Autodesk Fusion 360 part; units mm, degrees
(part 2 of 11)
  spline S13 degree 5 poles (-14.6436, -12.9958) (-14.6439, -12.9989) (-14.6444, -13.005) (-14.6453, -13.0142) (-14.6463, -13.0265) (-14.6476, -13.0418) (-14.6488, -13.0571) (-14.6499, -13.0724) (-14.6509, -13.0877) (-14.6519, -13.1029) (-14.6528, -13.1182) (-14.6536, -13.1334) (-14.6544, -13.1486) (-14.6551, -13.1638) (-14.6557, -13.1789) (-14.6562, -13.194) (-14.6567, -13.2091) (-14.6571, -13.2242) (-14.6574, -13.2393) (-14.6577, -13.2543) (-14.6579, -13.2693) (-14.658, -13.2843) (-14.658, -13.2993) (-14.658, -13.3142) (-14.6578, -13.3291) (-14.6577, -13.344) (-14.6574, -13.3589) (-14.657, -13.3737) (-14.6566, -13.3886) (-14.6561, -13.4033) (-14.6555, -13.4181) (-14.6549, -13.4328) (-14.6541, -13.4475) (-14.6533, -13.4622) (-14.6524, -13.4768) (-14.6514, -13.4915) (-14.6504, -13.506) (-14.6492, -13.5206) (-14.648, -13.5351) (-14.6467, -13.5496) (-14.6453, -13.564) (-14.6438, -13.5785) (-14.6422, -13.5928) (-14.6405, -13.6072) (-14.6388, -13.6215) (-14.637, -13.6358) (-14.635, -13.65) (-14.633, -13.6642) (-14.6309, -13.6784) (-14.6287, -13.6925) (-14.6264, -13.7066) (-14.624, -13.7206) (-14.6215, -13.7346) (-14.6188, -13.7486) (-14.6161, -13.7625) (-14.6133, -13.7763) (-14.6103, -13.7902) (-14.6073, -13.8039) (-14.6042, -13.8177) (-14.601, -13.8313) (-14.5976, -13.8449) (-14.5941, -13.8585) (-14.5903, -13.8719) (-14.5865, -13.8853) (-14.5825, -13.8986) (-14.5783, -13.9119) (-14.5741, -13.9251) (-14.5699, -13.9383) (-14.5654, -13.9514) (-14.5608, -13.9644) (-14.5558, -13.9772) (-14.5515, -13.9873) (-14.5479, -13.9947) (-14.5455, -13.9996) (-14.5442, -14.0021) knots -1 -1 -1 -1 -1 -1 -0.98571429 -0.97142857 -0.95714286 -0.94285714 -0.92857143 -0.91428571 -0.9 -0.88571429 -0.87142857 -0.85714286 -0.84285714 -0.82857143 -0.81428571 -0.8 -0.78571429 -0.77142857 -0.75714286 -0.74285714 -0.72857143 -0.71428571 -0.7 -0.68571429 -0.67142857 -0.65714286 -0.64285714 -0.62857143 -0.61428571 -0.6 -0.58571429 -0.57142857 -0.55714286 -0.54285714 -0.52857143 -0.51428571 -0.5 -0.48571429 -0.47142857 -0.45714286 -0.44285714 -0.42857143 -0.41428571 -0.4 -0.38571429 -0.37142857 -0.35714286 -0.34285714 -0.32857143 -0.31428571 -0.3 -0.28571429 -0.27142857 -0.25714286 -0.24285714 -0.22857143 -0.21428571 -0.2 -0.18571429 -0.17142857 -0.15714286 -0.14285714 -0.12857143 -0.11428571 -0.1 -0.08571429 -0.07142857 -0.05714286 -0.04285714 -0.02857143 -0.01428571 0 0 0 0 0 0
  line L13 (-14.5442, -14.0021) -> (-14.5127, -14.0629)
  arc A27 (-14.6099, -14.3947) -> (-14.5127, -14.0629) centre (-14.7346, -14.178) ccw
  arc A28 (-14.6099, -14.3947) -> (-14.7093, -14.4532) centre (-11.6741, -19.5) ccw
  arc A29 (-15.0466, -14.3769) -> (-14.7093, -14.4532) centre (-14.8381, -14.2389) ccw
  line L14 (-15.0466, -14.3769) -> (-15.0844, -14.3198)
  spline S14 degree 5 poles (-15.0844, -14.3198) (-15.0859, -14.3175) (-15.089, -14.313) (-15.0938, -14.3062) (-15.1005, -14.2975) (-15.1093, -14.287) (-15.1184, -14.2766) (-15.1277, -14.2664) (-15.1371, -14.2562) (-15.1466, -14.2461) (-15.1562, -14.2361) (-15.1659, -14.2261) (-15.1757, -14.2162) (-15.1857, -14.2064) (-15.1958, -14.1968) (-15.206, -14.1872) (-15.2164, -14.1777) (-15.2269, -14.1683) (-15.2375, -14.159) (-15.2481, -14.1497) (-15.2589, -14.1405) (-15.2697, -14.1314) (-15.2806, -14.1223) (-15.2916, -14.1133) (-15.3027, -14.1044) (-15.3139, -14.0955) (-15.3252, -14.0867) (-15.3365, -14.078) (-15.3479, -14.0693) (-15.3594, -14.0607) (-15.371, -14.0522) (-15.3827, -14.0437) (-15.3944, -14.0353) (-15.4062, -14.0269) (-15.4181, -14.0186) (-15.4301, -14.0103) (-15.4421, -14.0022) (-15.4542, -13.994) (-15.4663, -13.9859) (-15.4786, -13.9779) (-15.4909, -13.97) (-15.5032, -13.9621) (-15.5156, -13.9542) (-15.5281, -13.9464) (-15.5407, -13.9387) (-15.5533, -13.931) (-15.566, -13.9234) (-15.5787, -13.9158) (-15.5915, -13.9083) (-15.6044, -13.9008) (-15.6173, -13.8934) (-15.6303, -13.8861) (-15.6433, -13.8788) (-15.6564, -13.8715) (-15.6696, -13.8643) (-15.6828, -13.8572) (-15.696, -13.8501) (-15.7093, -13.8431) (-15.7227, -13.8361) (-15.7362, -13.8292) (-15.7496, -13.8223) (-15.7632, -13.8155) (-15.7768, -13.8087) (-15.7904, -13.802) (-15.8041, -13.7953) (-15.8179, -13.7887) (-15.8317, -13.7822) (-15.8455, -13.7757) (-15.8594, -13.7692) (-15.8734, -13.7628) (-15.8874, -13.7564) (-15.8986, -13.7514) (-15.9071, -13.7476) (-15.9127, -13.7451) (-15.9156, -13.7439) knots 0 0 0 0 0 0 0.01428571 0.02857143 0.04285714 0.05714286 0.07142857 0.08571429 0.1 0.11428571 0.12857143 0.14285714 0.15714286 0.17142857 0.18571429 0.2 0.21428571 0.22857143 0.24285714 0.25714286 0.27142857 0.28571429 0.3 0.31428571 0.32857143 0.34285714 0.35714286 0.37142857 0.38571429 0.4 0.41428571 0.42857143 0.44285714 0.45714286 0.47142857 0.48571429 0.5 0.51428571 0.52857143 0.54285714 0.55714286 0.57142857 0.58571429 0.6 0.61428571 0.62857143 0.64285714 0.65714286 0.67142857 0.68571429 0.7 0.71428571 0.72857143 0.74285714 0.75714286 0.77142857 0.78571429 0.8 0.81428571 0.82857143 0.84285714 0.85714286 0.87142857 0.88571429 0.9 0.91428571 0.92857143 0.94285714 0.95714286 0.97142857 0.98571429 1 1 1 1 1 1
  arc A30 (-15.9156, -13.7439) -> (-16.2258, -13.986) centre (-11.6741, -19.5) ccw
  spline S15 degree 5 poles (-16.2258, -13.986) (-16.2253, -13.989) (-16.2243, -13.9951) (-16.2227, -14.0042) (-16.2205, -14.0163) (-16.2178, -14.0315) (-16.2149, -14.0466) (-16.2121, -14.0616) (-16.2091, -14.0766) (-16.2061, -14.0916) (-16.203, -14.1066) (-16.1999, -14.1215) (-16.1967, -14.1363) (-16.1934, -14.1512) (-16.1901, -14.166) (-16.1867, -14.1807) (-16.1833, -14.1954) (-16.1798, -14.2101) (-16.1762, -14.2247) (-16.1725, -14.2393) (-16.1688, -14.2539) (-16.165, -14.2684) (-16.1612, -14.2829) (-16.1573, -14.2973) (-16.1533, -14.3117) (-16.1493, -14.326) (-16.1452, -14.3403) (-16.141, -14.3545) (-16.1367, -14.3687) (-16.1324, -14.3829) (-16.128, -14.397) (-16.1236, -14.411) (-16.1191, -14.425) (-16.1145, -14.439) (-16.1098, -14.4529) (-16.1051, -14.4668) (-16.1003, -14.4806) (-16.0954, -14.4943) (-16.0905, -14.508) (-16.0855, -14.5217) (-16.0804, -14.5353) (-16.0752, -14.5488) (-16.07, -14.5623) (-16.0646, -14.5757) (-16.0592, -14.5891) (-16.0538, -14.6024) (-16.0482, -14.6157) (-16.0426, -14.6289) (-16.0369, -14.642) (-16.0311, -14.6551) (-16.0252, -14.6681) (-16.0193, -14.681) (-16.0132, -14.6939) (-16.0071, -14.7067) (-16.0008, -14.7194) (-15.9945, -14.7321) (-15.9881, -14.7447) (-15.9816, -14.7572) (-15.9751, -14.7696) (-15.9684, -14.782) (-15.9616, -14.7943) (-15.9547, -14.8064) (-15.9476, -14.8185) (-15.9404, -14.8304) (-15.9331, -14.8422) (-15.9257, -14.854) (-15.9182, -14.8656) (-15.9107, -14.8772) (-15.903, -14.8888) (-15.8952, -14.9001) (-15.887, -14.9112) (-15.8802, -14.9198) (-15.8749, -14.9261) (-15.8712, -14.9302) (-15.8694, -14.9322) knots -1 -1 -1 -1 -1 -1 -0.98571429 -0.97142857 -0.95714286 -0.94285714 -0.92857143 -0.91428571 -0.9 -0.88571429 -0.87142857 -0.85714286 -0.84285714 -0.82857143 -0.81428571 -0.8 -0.78571429 -0.77142857 -0.75714286 -0.74285714 -0.72857143 -0.71428571 -0.7 -0.68571429 -0.67142857 -0.65714286 -0.64285714 -0.62857143 -0.61428571 -0.6 -0.58571429 -0.57142857 -0.55714286 -0.54285714 -0.52857143 -0.51428571 -0.5 -0.48571429 -0.47142857 -0.45714286 -0.44285714 -0.42857143 -0.41428571 -0.4 -0.38571429 -0.37142857 -0.35714286 -0.34285714 -0.32857143 -0.31428571 -0.3 -0.28571429 -0.27142857 -0.25714286 -0.24285714 -0.22857143 -0.21428571 -0.2 -0.18571429 -0.17142857 -0.15714286 -0.14285714 -0.12857143 -0.11428571 -0.1 -0.08571429 -0.07142857 -0.05714286 -0.04285714 -0.02857143 -0.01428571 0 0 0 0 0 0
  line L15 (-15.8694, -14.9322) -> (-15.8232, -14.9828)
  arc A31 (-15.8312, -15.3285) -> (-15.8232, -14.9828) centre (-16.0077, -15.1515) ccw
  arc A32 (-15.8312, -15.3285) -> (-15.9121, -15.4107) centre (-11.6741, -19.5) ccw
  arc A33 (-16.2576, -15.4243) -> (-15.9121, -15.4107) centre (-16.092, -15.2371) ccw
  line L16 (-16.2576, -15.4243) -> (-16.3089, -15.3789)
  spline S16 degree 5 poles (-16.3089, -15.3789) (-16.311, -15.3771) (-16.3151, -15.3735) (-16.3215, -15.3683) (-16.3302, -15.3616) (-16.3415, -15.3537) (-16.3529, -15.346) (-16.3646, -15.3385) (-16.3763, -15.3312) (-16.3881, -15.3239) (-16.4, -15.3167) (-16.4119, -15.3095) (-16.424, -15.3025) (-16.4361, -15.2957) (-16.4484, -15.2889) (-16.4608, -15.2823) (-16.4732, -15.2759) (-16.4858, -15.2695) (-16.4984, -15.2632) (-16.5111, -15.257) (-16.5238, -15.2509) (-16.5367, -15.2449) (-16.5496, -15.239) (-16.5625, -15.2331) (-16.5755, -15.2274) (-16.5886, -15.2217) (-16.6018, -15.2161) (-16.615, -15.2106) (-16.6283, -15.2052) (-16.6417, -15.1999) (-16.6551, -15.1946) (-16.6685, -15.1894) (-16.682, -15.1843) (-16.6956, -15.1793) (-16.7092, -15.1744) (-16.7229, -15.1695) (-16.7366, -15.1647) (-16.7504, -15.16) (-16.7643, -15.1553) (-16.7781, -15.1508) (-16.7921, -15.1462) (-16.8061, -15.1418) (-16.8201, -15.1374) (-16.8342, -15.1332) (-16.8483, -15.1289) (-16.8625, -15.1248) (-16.8767, -15.1207) (-16.891, -15.1167) (-16.9053, -15.1127) (-16.9196, -15.1089) (-16.934, -15.105) (-16.9485, -15.1013) (-16.9629, -15.0976) (-16.9775, -15.094) (-16.992, -15.0905) (-17.0066, -15.087) (-17.0213, -15.0836) (-17.036, -15.0802) (-17.0507, -15.077) (-17.0655, -15.0737) (-17.0803, -15.0706) (-17.0951, -15.0675) (-17.11, -15.0645) (-17.1249, -15.0615) (-17.1399, -15.0586) (-17.1549, -15.0558) (-17.1699, -15.053) (-17.185, -15.0503) (-17.2001, -15.0477) (-17.2152, -15.0451) (-17.2304, -15.0426) (-17.2425, -15.0407) (-17.2517, -15.0392) (-17.2578, -15.0383) (-17.2608, -15.0378) knots 0 0 0 0 0 0 0.01428571 0.02857143 0.04285714 0.05714286 0.07142857 0.08571429 0.1 0.11428571 0.12857143 0.14285714 0.15714286 0.17142857 0.18571429 0.2 0.21428571 0.22857143 0.24285714 0.25714286 0.27142857 0.28571429 0.3 0.31428571 0.32857143 0.34285714 0.35714286 0.37142857 0.38571429 0.4 0.41428571 0.42857143 0.44285714 0.45714286 0.47142857 0.48571429 0.5 0.51428571 0.52857143 0.54285714 0.55714286 0.57142857 0.58571429 0.6 0.61428571 0.62857143 0.64285714 0.65714286 0.67142857 0.68571429 0.7 0.71428571 0.72857143 0.74285714 0.75714286 0.77142857 0.78571429 0.8 0.81428571 0.82857143 0.84285714 0.85714286 0.87142857 0.88571429 0.9 0.91428571 0.92857143 0.94285714 0.95714286 0.97142857 0.98571429 1 1 1 1 1 1
  arc A34 (-17.2608, -15.0378) -> (-17.4979, -15.3519) centre (-11.6741, -19.5) ccw
  spline S17 degree 5 poles (-17.4979, -15.3519) (-17.4966, -15.3547) (-17.494, -15.3603) (-17.4901, -15.3687) (-17.4849, -15.3799) (-17.4783, -15.3938) (-17.4717, -15.4076) (-17.465, -15.4214) (-17.4583, -15.4352) (-17.4515, -15.4489) (-17.4446, -15.4625) (-17.4378, -15.4761) (-17.4308, -15.4896) (-17.4238, -15.5031) (-17.4168, -15.5165) (-17.4097, -15.5299) (-17.4026, -15.5432) (-17.3954, -15.5565) (-17.3881, -15.5697) (-17.3808, -15.5829) (-17.3735, -15.5959) (-17.3661, -15.609) (-17.3586, -15.622) (-17.3511, -15.6349) (-17.3435, -15.6477) (-17.3359, -15.6605) (-17.3283, -15.6733) (-17.3205, -15.6859) (-17.3128, -15.6986) (-17.3049, -15.7111) (-17.297, -15.7236) (-17.2891, -15.736) (-17.2811, -15.7484) (-17.2731, -15.7607) (-17.265, -15.7729) (-17.2568, -15.7851) (-17.2486, -15.7972) (-17.2403, -15.8092) (-17.232, -15.8212) (-17.2236, -15.8331) (-17.2152, -15.8449) (-17.2067, -15.8566) (-17.1981, -15.8683) (-17.1895, -15.8799) (-17.1809, -15.8914) (-17.1721, -15.9028) (-17.1633, -15.9142) (-17.1545, -15.9255) (-17.1456, -15.9367) (-17.1366, -15.9478) (-17.1276, -15.9589) (-17.1184, -15.9698) (-17.1093, -15.9807) (-17.1, -15.9915) (-17.0907, -16.0021) (-17.0813, -16.0127) (-17.0719, -16.0232) (-17.0624, -16.0336) (-17.0528, -16.044) (-17.0432, -16.0542) (-17.0335, -16.0643) (-17.0236, -16.0742) (-17.0137, -16.084) (-17.0036, -16.0937) (-16.9935, -16.1032) (-16.9833, -16.1126) (-16.9731, -16.122) (-16.9628, -16.1313) (-16.9524, -16.1404) (-16.9419, -16.1493) (-16.9312, -16.158) (-16.9223, -16.1645) (-16.9156, -16.1692) (-16.911, -16.1722) (-16.9087, -16.1737) knots -1 -1 -1 -1 -1 -1 -0.98571429 -0.97142857 -0.95714286 -0.94285714 -0.92857143 -0.91428571 -0.9 -0.88571429 -0.87142857 -0.85714286 -0.84285714 -0.82857143 -0.81428571 -0.8 -0.78571429 -0.77142857 -0.75714286 -0.74285714 -0.72857143 -0.71428571 -0.7 -0.68571429 -0.67142857 -0.65714286 -0.64285714 -0.62857143 -0.61428571 -0.6 -0.58571429 -0.57142857 -0.55714286 -0.54285714 -0.52857143 -0.51428571 -0.5 -0.48571429 -0.47142857 -0.45714286 -0.44285714 -0.42857143 -0.41428571 -0.4 -0.38571429 -0.37142857 -0.35714286 -0.34285714 -0.32857143 -0.31428571 -0.3 -0.28571429 -0.27142857 -0.25714286 -0.24285714 -0.22857143 -0.21428571 -0.2 -0.18571429 -0.17142857 -0.15714286 -0.14285714 -0.12857143 -0.11428571 -0.1 -0.08571429 -0.07142857 -0.05714286 -0.04285714 -0.02857143 -0.01428571 0 0 0 0 0 0
  line L17 (-16.9087, -16.1737) -> (-16.8509, -16.2106)
  arc A35 (-16.7692, -16.5466) -> (-16.8509, -16.2106) centre (-16.9855, -16.4212) ccw
  arc A36 (-16.7692, -16.5466) -> (-16.8261, -16.6469) centre (-11.6741, -19.5) ccw
  arc A37 (-17.1563, -16.7495) -> (-16.8261, -16.6469) centre (-17.0448, -16.5258) ccw
  line L18 (-17.1563, -16.7495) -> (-17.2176, -16.7189)
  spline S18 degree 5 poles (-17.2176, -16.7189) (-17.2201, -16.7177) (-17.225, -16.7153) (-17.2325, -16.7119) (-17.2427, -16.7077) (-17.2556, -16.7029) (-17.2687, -16.6985) (-17.2818, -16.6943) (-17.2951, -16.6902) (-17.3083, -16.6863) (-17.3217, -16.6823) (-17.3351, -16.6785) (-17.3485, -16.6749) (-17.362, -16.6714) (-17.3756, -16.6681) (-17.3893, -16.6649) (-17.403, -16.6619) (-17.4168, -16.659) (-17.4306, -16.6562) (-17.4444, -16.6535) (-17.4583, -16.6509) (-17.4723, -16.6484) (-17.4863, -16.646) (-17.5003, -16.6437) (-17.5144, -16.6415) (-17.5285, -16.6395) (-17.5426, -16.6375) (-17.5568, -16.6356) (-17.5711, -16.6338) (-17.5854, -16.6321) (-17.5997, -16.6305) (-17.614, -16.629) (-17.6284, -16.6275) (-17.6428, -16.6262) (-17.6572, -16.6249) (-17.6717, -16.6238) (-17.6862, -16.6227) (-17.7007, -16.6217) (-17.7153, -16.6208) (-17.7299, -16.62) (-17.7445, -16.6192) (-17.7592, -16.6186) (-17.7739, -16.618) (-17.7886, -16.6175) (-17.8033, -16.617) (-17.8181, -16.6167) (-17.8329, -16.6164) (-17.8477, -16.6162) (-17.8625, -16.6161) (-17.8774, -16.6161) (-17.8923, -16.6162) (-17.9072, -16.6163) (-17.9221, -16.6165) (-17.9371, -16.6167) (-17.9521, -16.6171) (-17.9671, -16.6175) (-17.9821, -16.618) (-17.9972, -16.6186) (-18.0123, -16.6192) (-18.0274, -16.6199) (-18.0425, -16.6207) (-18.0576, -16.6216) (-18.0728, -16.6225) (-18.0879, -16.6235) (-18.1031, -16.6246) (-18.1184, -16.6258) (-18.1336, -16.627) (-18.1488, -16.6283) (-18.1641, -16.6296) (-18.1794, -16.6311) (-18.1947, -16.6326) (-18.207, -16.6338) (-18.2162, -16.6348) (-18.2223, -16.6355) (-18.2254, -16.6358) knots 0 0 0 0 0 0 0.01428571 0.02857143 0.04285714 0.05714286 0.07142857 0.08571429 0.1 0.11428571 0.12857143 0.14285714 0.15714286 0.17142857 0.18571429 0.2 0.21428571 0.22857143 0.24285714 0.25714286 0.27142857 0.28571429 0.3 0.31428571 0.32857143 0.34285714 0.35714286 0.37142857 0.38571429 0.4 0.41428571 0.42857143 0.44285714 0.45714286 0.47142857 0.48571429 0.5 0.51428571 0.52857143 0.54285714 0.55714286 0.57142857 0.58571429 0.6 0.61428571 0.62857143 0.64285714 0.65714286 0.67142857 0.68571429 0.7 0.71428571 0.72857143 0.74285714 0.75714286 0.77142857 0.78571429 0.8 0.81428571 0.82857143 0.84285714 0.85714286 0.87142857 0.88571429 0.9 0.91428571 0.92857143 0.94285714 0.95714286 0.97142857 0.98571429 1 1 1 1 1 1
  arc A38 (-18.2254, -16.6358) -> (-18.373, -17.0005) centre (-11.6741, -19.5) ccw
  spline S19 degree 5 poles (-18.373, -17.0005) (-18.3711, -17.0029) (-18.3671, -17.0077) (-18.3612, -17.0148) (-18.3532, -17.0242) (-18.3433, -17.0359) (-18.3333, -17.0476) (-18.3233, -17.0592) (-18.3132, -17.0707) (-18.3031, -17.0822) (-18.293, -17.0936) (-18.2828, -17.1049) (-18.2726, -17.1162) (-18.2624, -17.1274) (-18.2521, -17.1386) (-18.2418, -17.1497) (-18.2314, -17.1607) (-18.2211, -17.1716) (-18.2106, -17.1825) (-18.2002, -17.1933) (-18.1897, -17.2041) (-18.1792, -17.2147) (-18.1686, -17.2253) (-18.158, -17.2359) (-18.1474, -17.2463) (-18.1367, -17.2567) (-18.126, -17.2671) (-18.1153, -17.2773) (-18.1045, -17.2875) (-18.0937, -17.2976) (-18.0829, -17.3076) (-18.072, -17.3175) (-18.0611, -17.3274) (-18.0501, -17.3372) (-18.0391, -17.3469) (-18.0281, -17.3566) (-18.017, -17.3661) (-18.0059, -17.3756) (-17.9948, -17.385) (-17.9836, -17.3943) (-17.9724, -17.4036) (-17.9612, -17.4127) (-17.9499, -17.4218) (-17.9385, -17.4307) (-17.9272, -17.4396) (-17.9158, -17.4484) (-17.9044, -17.4571) (-17.8929, -17.4657) (-17.8814, -17.4742) (-17.8698, -17.4827) (-17.8582, -17.491) (-17.8466, -17.4992) (-17.8349, -17.5073) (-17.8232, -17.5153) (-17.8115, -17.5232) (-17.7997, -17.531) (-17.7878, -17.5387) (-17.7759, -17.5463) (-17.764, -17.5538) (-17.7521, -17.5612) (-17.7401, -17.5685) (-17.728, -17.5755) (-17.7159, -17.5824) (-17.7037, -17.5891) (-17.6914, -17.5957) (-17.6791, -17.6022) (-17.6668, -17.6086) (-17.6545, -17.6148) (-17.6421, -17.621) (-17.6296, -17.6269) (-17.617, -17.6325) (-17.6068, -17.6365) (-17.599, -17.6393) (-17.5938, -17.641) (-17.5912, -17.6418) knots -1 -1 -1 -1 -1 -1 -0.98571429 -0.97142857 -0.95714286 -0.94285714 -0.92857143 -0.91428571 -0.9 -0.88571429 -0.87142857 -0.85714286 -0.84285714 -0.82857143 -0.81428571 -0.8 -0.78571429 -0.77142857 -0.75714286 -0.74285714 -0.72857143 -0.71428571 -0.7 -0.68571429 -0.67142857 -0.65714286 -0.64285714 -0.62857143 -0.61428571 -0.6 -0.58571429 -0.57142857 -0.55714286 -0.54285714 -0.52857143 -0.51428571 -0.5 -0.48571429 -0.47142857 -0.45714286 -0.44285714 -0.42857143 -0.41428571 -0.4 -0.38571429 -0.37142857 -0.35714286 -0.34285714 -0.32857143 -0.31428571 -0.3 -0.28571429 -0.27142857 -0.25714286 -0.24285714 -0.22857143 -0.21428571 -0.2 -0.18571429 -0.17142857 -0.15714286 -0.14285714 -0.12857143 -0.11428571 -0.1 -0.08571429 -0.07142857 -0.05714286 -0.04285714 -0.02857143 -0.01428571 0 0 0 0 0 0
  line L19 (-17.5912, -17.6418) -> (-17.5259, -17.6625)
  arc A39 (-17.36, -17.966) -> (-17.5259, -17.6625) centre (-17.6014, -17.9008) ccw
  arc A40 (-17.36, -17.966) -> (-17.389, -18.0775) centre (-11.6741, -19.5) ccw
  arc A41 (-17.6814, -18.2621) -> (-17.389, -18.0775) centre (-17.6316, -18.0171) ccw
  line L20 (-17.6814, -18.2621) -> (-17.7485, -18.2485)
  spline S20 degree 5 poles (-17.7485, -18.2485) (-17.7512, -18.2479) (-17.7566, -18.2469) (-17.7647, -18.2455) (-17.7756, -18.2441) (-17.7893, -18.2428) (-17.8031, -18.2419) (-17.8169, -18.2413) (-17.8308, -18.2408) (-17.8446, -18.2404) (-17.8585, -18.24) (-17.8724, -18.2398) (-17.8863, -18.2398) (-17.9003, -18.2399) (-17.9143, -18.2402) (-17.9283, -18.2407) (-17.9423, -18.2414) (-17.9564, -18.2421) (-17.9705, -18.243) (-17.9845, -18.244) (-17.9986, -18.245) (-18.0128, -18.2462) (-18.0269, -18.2475) (-18.041, -18.249) (-18.0552, -18.2505) (-18.0694, -18.2521) (-18.0836, -18.2539) (-18.0978, -18.2558) (-18.112, -18.2577) (-18.1262, -18.2598) (-18.1404, -18.2619) (-18.1547, -18.2641) (-18.1689, -18.2665) (-18.1832, -18.2689) (-18.1975, -18.2714) (-18.2118, -18.2741) (-18.226, -18.2768) (-18.2403, -18.2796) (-18.2547, -18.2825) (-18.269, -18.2854) (-18.2833, -18.2885) (-18.2976, -18.2917) (-18.3119, -18.2949) (-18.3263, -18.2982) (-18.3406, -18.3016) (-18.355, -18.3051) (-18.3693, -18.3087) (-18.3837, -18.3123) (-18.3981, -18.3161) (-18.4124, -18.3199) (-18.4268, -18.3238) (-18.4412, -18.3278) (-18.4556, -18.3318) (-18.4699, -18.336) (-18.4843, -18.3402) (-18.4987, -18.3445) (-18.5131, -18.3488) (-18.5275, -18.3533) (-18.5419, -18.3578) (-18.5563, -18.3624) (-18.5707, -18.3671) (-18.5851, -18.3718) (-18.5995, -18.3767) (-18.6139, -18.3816) (-18.6283, -18.3865) (-18.6427, -18.3916) (-18.6571, -18.3967) (-18.6715, -18.4019) (-18.6859, -18.4072) (-18.7003, -18.4125) (-18.7147, -18.4179) (-18.7262, -18.4223) (-18.7348, -18.4256) (-18.7406, -18.4278) (-18.7435, -18.429) knots 0 0 0 0 0 0 0.01428571 0.02857143 0.04285714 0.05714286 0.07142857 0.08571429 0.1 0.11428571 0.12857143 0.14285714 0.15714286 0.17142857 0.18571429 0.2 0.21428571 0.22857143 0.24285714 0.25714286 0.27142857 0.28571429 0.3 0.31428571 0.32857143 0.34285714 0.35714286 0.37142857 0.38571429 0.4 0.41428571 0.42857143 0.44285714 0.45714286 0.47142857 0.48571429 0.5 0.51428571 0.52857143 0.54285714 0.55714286 0.57142857 0.58571429 0.6 0.61428571 0.62857143 0.64285714 0.65714286 0.67142857 0.68571429 0.7 0.71428571 0.72857143 0.74285714 0.75714286 0.77142857 0.78571429 0.8 0.81428571 0.82857143 0.84285714 0.85714286 0.87142857 0.88571429 0.9 0.91428571 0.92857143 0.94285714 0.95714286 0.97142857 0.98571429 1 1 1 1 1 1
  arc A42 (-18.7435, -18.429) -> (-18.7917, -18.8195) centre (-11.6741, -19.5) ccw
  spline S21 degree 5 poles (-18.7917, -18.8195) (-18.7892, -18.8213) (-18.7841, -18.8249) (-18.7766, -18.8302) (-18.7664, -18.8372) (-18.7538, -18.846) (-18.7411, -18.8547) (-18.7284, -18.8633) (-18.7157, -18.8718) (-18.703, -18.8803) (-18.6903, -18.8887) (-18.6775, -18.897) (-18.6647, -18.9053) (-18.652, -18.9134) (-18.6391, -18.9216) (-18.6263, -18.9296) (-18.6135, -18.9376) (-18.6006, -18.9454) (-18.5877, -18.9533) (-18.5748, -18.961) (-18.5619, -18.9687) (-18.549, -18.9762) (-18.536, -18.9838) (-18.5231, -18.9912) (-18.5101, -18.9985) (-18.4971, -19.0058) (-18.4841, -19.013) (-18.4711, -19.0201) (-18.458, -19.0272) (-18.445, -19.0341) (-18.4319, -19.041) (-18.4188, -19.0478) (-18.4057, -19.0545) (-18.3926, -19.0611) (-18.3795, -19.0677) (-18.3663, -19.0741) (-18.3532, -19.0805) (-18.34, -19.0868) (-18.3268, -19.093) (-18.3136, -19.0991) (-18.3004, -19.1051) (-18.2872, -19.111) (-18.2739, -19.1168) (-18.2607, -19.1226) (-18.2474, -19.1282) (-18.2341, -19.1338) (-18.2208, -19.1392) (-18.2075, -19.1446) (-18.1942, -19.1498) (-18.1808, -19.155) (-18.1675, -19.16) (-18.1541, -19.165) (-18.1407, -19.1698) (-18.1274, -19.1745) (-18.114, -19.1791) (-18.1005, -19.1835) (-18.0871, -19.1879) (-18.0737, -19.1922) (-18.0602, -19.1963) (-18.0468, -19.2004) (-18.0333, -19.2042) (-18.0198, -19.208) (-18.0063, -19.2115) (-17.9928, -19.2148) (-17.9792, -19.218) (-17.9657, -19.2211) (-17.9521, -19.224) (-17.9386, -19.2269) (-17.925, -19.2296) (-17.9115, -19.2321) (-17.8979, -19.2342) (-17.887, -19.2355) (-17.8787, -19.2362) (-17.8733, -19.2365) (-17.8705, -19.2366) knots -1 -1 -1 -1 -1 -1 -0.98571429 -0.97142857 -0.95714286 -0.94285714 -0.92857143 -0.91428571 -0.9 -0.88571429 -0.87142857 -0.85714286 -0.84285714 -0.82857143 -0.81428571 -0.8 -0.78571429 -0.77142857 -0.75714286 -0.74285714 -0.72857143 -0.71428571 -0.7 -0.68571429 -0.67142857 -0.65714286 -0.64285714 -0.62857143 -0.61428571 -0.6 -0.58571429 -0.57142857 -0.55714286 -0.54285714 -0.52857143 -0.51428571 -0.5 -0.48571429 -0.47142857 -0.45714286 -0.44285714 -0.42857143 -0.41428571 -0.4 -0.38571429 -0.37142857 -0.35714286 -0.34285714 -0.32857143 -0.31428571 -0.3 -0.28571429 -0.27142857 -0.25714286 -0.24285714 -0.22857143 -0.21428571 -0.2 -0.18571429 -0.17142857 -0.15714286 -0.14285714 -0.12857143 -0.11428571 -0.1 -0.08571429 -0.07142857 -0.05714286 -0.04285714 -0.02857143 -0.01428571 0 0 0 0 0 0
  line L21 (-17.8705, -19.2366) -> (-17.8021, -19.2397)
  arc A43 (-17.5633, -19.4898) -> (-17.8021, -19.2397) centre (-17.8133, -19.4894) ccw
  arc A44 (-17.5633, -19.4898) -> (-17.5624, -19.6051) centre (-11.6741, -19.5) ccw
  arc A45 (-17.7971, -19.8591) -> (-17.5624, -19.6051) centre (-17.8124, -19.6095) ccw
  line L22 (-17.7971, -19.8591) -> (-17.8655, -19.8633)
  spline S22 degree 5 poles (-17.8655, -19.8633) (-17.8682, -19.8634) (-17.8737, -19.8638) (-17.8819, -19.8646) (-17.8928, -19.8661) (-17.9063, -19.8684) (-17.9199, -19.8711) (-17.9334, -19.8741) (-17.9469, -19.8771) (-17.9604, -19.8803) (-17.9739, -19.8836) (-17.9874, -19.887) (-18.0008, -19.8906) (-18.0143, -19.8943) (-18.0277, -19.8982) (-18.0411, -19.9023) (-18.0545, -19.9066) (-18.0679, -19.9109) (-18.0813, -19.9154) (-18.0946, -19.92) (-18.1079, -19.9247) (-18.1213, -19.9295) (-18.1346, -19.9344) (-18.1479, -19.9395) (-18.1612, -19.9446) (-18.1744, -19.9499) (-18.1877, -19.9552) (-18.2009, -19.9607) (-18.2141, -19.9663) (-18.2273, -19.9719) (-18.2405, -19.9777) (-18.2537, -19.9835) (-18.2669, -19.9895) (-18.28, -19.9955) (-18.2932, -20.0017) (-18.3063, -20.0079) (-18.3194, -20.0142) (-18.3325, -20.0206) (-18.3455, -20.0271) (-18.3586, -20.0337) (-18.3716, -20.0404) (-18.3847, -20.0471) (-18.3977, -20.0539) (-18.4107, -20.0609) (-18.4236, -20.0679) (-18.4366, -20.075) (-18.4495, -20.0821) (-18.4625, -20.0894) (-18.4754, -20.0967) (-18.4883, -20.1041) (-18.5011, -20.1116) (-18.514, -20.1192) (-18.5268, -20.1268) (-18.5397, -20.1345) (-18.5525, -20.1423) (-18.5653, -20.1502) (-18.578, -20.1581) (-18.5908, -20.1661) (-18.6035, -20.1742) (-18.6162, -20.1824) (-18.6289, -20.1906) (-18.6416, -20.199) (-18.6543, -20.2073) (-18.6669, -20.2158) (-18.6795, -20.2243) (-18.6921, -20.2329) (-18.7047, -20.2416) (-18.7173, -20.2504) (-18.7298, -20.2592) (-18.7423, -20.2681) (-18.7548, -20.277) (-18.7648, -20.2842) (-18.7723, -20.2897) (-18.7773, -20.2933) (-18.7798, -20.2951) knots 0 0 0 0 0 0 0.01428571 0.02857143 0.04285714 0.05714286 0.07142857 0.08571429 0.1 0.11428571 0.12857143 0.14285714 0.15714286 0.17142857 0.18571429 0.2 0.21428571 0.22857143 0.24285714 0.25714286 0.27142857 0.28571429 0.3 0.31428571 0.32857143 0.34285714 0.35714286 0.37142857 0.38571429 0.4 0.41428571 0.42857143 0.44285714 0.45714286 0.47142857 0.48571429 0.5 0.51428571 0.52857143 0.54285714 0.55714286 0.57142857 0.58571429 0.6 0.61428571 0.62857143 0.64285714 0.65714286 0.67142857 0.68571429 0.7 0.71428571 0.72857143 0.74285714 0.75714286 0.77142857 0.78571429 0.8 0.81428571 0.82857143 0.84285714 0.85714286 0.87142857 0.88571429 0.9 0.91428571 0.92857143 0.94285714 0.95714286 0.97142857 0.98571429 1 1 1 1 1 1
  arc A46 (-18.7798, -20.2951) -> (-18.7253, -20.6848) centre (-11.6741, -19.5) ccw
  spline S23 degree 5 poles (-18.7253, -20.6848) (-18.7224, -20.6859) (-18.7166, -20.6881) (-18.7079, -20.6912) (-18.6963, -20.6954) (-18.6818, -20.7006) (-18.6674, -20.7057) (-18.6529, -20.7108) (-18.6384, -20.7157) (-18.6239, -20.7206) (-18.6094, -20.7254) (-18.595, -20.7302) (-18.5805, -20.7348) (-18.566, -20.7394) (-18.5515, -20.7439) (-18.5371, -20.7484) (-18.5226, -20.7527) (-18.5081, -20.757) (-18.4937, -20.7613) (-18.4792, -20.7654) (-18.4648, -20.7694) (-18.4503, -20.7734) (-18.4359, -20.7773) (-18.4214, -20.7812) (-18.407, -20.7849) (-18.3925, -20.7886) (-18.3781, -20.7922) (-18.3637, -20.7957) (-18.3493, -20.7991) (-18.3349, -20.8024) (-18.3204, -20.8057) (-18.306, -20.8089) (-18.2917, -20.8119) (-18.2773, -20.815) (-18.2629, -20.8179) (-18.2485, -20.8207) (-18.2342, -20.8235) (-18.2198, -20.8261) (-18.2055, -20.8287) (-18.1911, -20.8312) (-18.1768, -20.8336) (-18.1625, -20.8358) (-18.1482, -20.8381) (-18.1339, -20.8402) (-18.1196, -20.8422) (-18.1054, -20.8441) (-18.0911, -20.8459) (-18.0769, -20.8476) (-18.0626, -20.8493) (-18.0484, -20.8508) (-18.0342, -20.8522) (-18.02, -20.8535) (-18.0059, -20.8547) (-17.9917, -20.8558) (-17.9776, -20.8567) (-17.9635, -20.8576) (-17.9494, -20.8583) (-17.9353, -20.859) (-17.9212, -20.8595) (-17.9072, -20.8599) (-17.8932, -20.8602) (-17.8792, -20.8603) (-17.8652, -20.8602) (-17.8513, -20.8599) (-17.8374, -20.8595) (-17.8235, -20.8589) (-17.8097, -20.8583) (-17.7958, -20.8576) (-17.782, -20.8567) (-17.7683, -20.8556) (-17.7546, -20.8541) (-17.7437, -20.8525) (-17.7356, -20.851) (-17.7302, -20.8499) (-17.7276, -20.8493) knots -1 -1 -1 -1 -1 -1 -0.98571429 -0.97142857 -0.95714286 -0.94285714 -0.92857143 -0.91428571 -0.9 -0.88571429 -0.87142857 -0.85714286 -0.84285714 -0.82857143 -0.81428571 -0.8 -0.78571429 -0.77142857 -0.75714286 -0.74285714 -0.72857143 -0.71428571 -0.7 -0.68571429 -0.67142857 -0.65714286 -0.64285714 -0.62857143 -0.61428571 -0.6 -0.58571429 -0.57142857 -0.55714286 -0.54285714 -0.52857143 -0.51428571 -0.5 -0.48571429 -0.47142857 -0.45714286 -0.44285714 -0.42857143 -0.41428571 -0.4 -0.38571429 -0.37142857 -0.35714286 -0.34285714 -0.32857143 -0.31428571 -0.3 -0.28571429 -0.27142857 -0.25714286 -0.24285714 -0.22857143 -0.21428571 -0.2 -0.18571429 -0.17142857 -0.15714286 -0.14285714 -0.12857143 -0.11428571 -0.1 -0.08571429 -0.07142857 -0.05714286 -0.04285714 -0.02857143 -0.01428571 0 0 0 0 0 0
  line L23 (-17.7276, -20.8493) -> (-17.6607, -20.8346)
  arc A47 (-17.3653, -21.0144) -> (-17.6607, -20.8346) centre (-17.6069, -21.0787) ccw
  arc A48 (-17.3653, -21.0144) -> (-17.3346, -21.1255) centre (-11.6741, -19.5) ccw
  arc A49 (-17.4955, -21.4316) -> (-17.3346, -21.1255) centre (-17.5749, -21.1945) ccw
  line L24 (-17.4955, -21.4316) -> (-17.5605, -21.4533)
  spline S24 degree 5 poles (-17.5605, -21.4533) (-17.5631, -21.4542) (-17.5683, -21.456) (-17.576, -21.4589) (-17.5861, -21.4631) (-17.5986, -21.4689) (-17.611, -21.475) (-17.6233, -21.4813) (-17.6355, -21.4878) (-17.6477, -21.4944) (-17.6599, -21.501) (-17.6721, -21.5078) (-17.6842, -21.5147) (-17.6962, -21.5218) (-17.7081, -21.5291) (-17.72, -21.5365) (-17.7319, -21.5441) (-17.7437, -21.5518) (-17.7554, -21.5596) (-17.7671, -21.5674) (-17.7788, -21.5754) (-17.7904, -21.5835) (-17.802, -21.5917) (-17.8136, -21.6) (-17.8251, -21.6084) (-17.8365, -21.6169) (-17.8479, -21.6256) (-17.8593, -21.6343) (-17.8706, -21.6431) (-17.8819, -21.6519) (-17.8932, -21.6609) (-17.9044, -21.67) (-17.9156, -21.6791) (-17.9267, -21.6884) (-17.9378, -21.6977) (-17.9488, -21.7071) (-17.9599, -21.7166) (-17.9709, -21.7262) (-17.9818, -21.7358) (-17.9927, -21.7456) (-18.0036, -21.7554) (-18.0144, -21.7653) (-18.0252, -21.7753) (-18.036, -21.7853) (-18.0467, -21.7954) (-18.0574, -21.8056) (-18.068, -21.8159) (-18.0786, -21.8262) (-18.0892, -21.8367) (-18.0997, -21.8471) (-18.1102, -21.8577) (-18.1207, -21.8683) (-18.1311, -21.879) (-18.1415, -21.8898) (-18.1518, -21.9007) (-18.1622, -21.9116) (-18.1724, -21.9226) (-18.1827, -21.9336) (-18.1929, -21.9447) (-18.2031, -21.9559) (-18.2132, -21.9671) (-18.2233, -21.9785) (-18.2333, -21.9898) (-18.2434, -22.0013) (-18.2533, -22.0128) (-18.2633, -22.0244) (-18.2732, -22.036) (-18.2831, -22.0477) (-18.2929, -22.0594) (-18.3027, -22.0713) (-18.3125, -22.0832) (-18.3202, -22.0927) (-18.3261, -22.0999) (-18.3299, -22.1047) (-18.3319, -22.1071) knots 0 0 0 0 0 0 0.01428571 0.02857143 0.04285714 0.05714286 0.07142857 0.08571429 0.1 0.11428571 0.12857143 0.14285714 0.15714286 0.17142857 0.18571429 0.2 0.21428571 0.22857143 0.24285714 0.25714286 0.27142857 0.28571429 0.3 0.31428571 0.32857143 0.34285714 0.35714286 0.37142857 0.38571429 0.4 0.41428571 0.42857143 0.44285714 0.45714286 0.47142857 0.48571429 0.5 0.51428571 0.52857143 0.54285714 0.55714286 0.57142857 0.58571429 0.6 0.61428571 0.62857143 0.64285714 0.65714286 0.67142857 0.68571429 0.7 0.71428571 0.72857143 0.74285714 0.75714286 0.77142857 0.78571429 0.8 0.81428571 0.82857143 0.84285714 0.85714286 0.87142857 0.88571429 0.9 0.91428571 0.92857143 0.94285714 0.95714286 0.97142857 0.98571429 1 1 1 1 1 1
  arc A50 (-18.3319, -22.1071) -> (-18.1784, -22.4694) centre (-11.6741, -19.5) ccw
  spline S25 degree 5 poles (-18.1784, -22.4694) (-18.1753, -22.4697) (-18.1691, -22.4703) (-18.1599, -22.4711) (-18.1476, -22.4722) (-18.1323, -22.4734) (-18.117, -22.4746) (-18.1017, -22.4757) (-18.0864, -22.4768) (-18.0712, -22.4777) (-18.056, -22.4787) (-18.0407, -22.4795) (-18.0256, -22.4802) (-18.0104, -22.4809) (-17.9952, -22.4816) (-17.9801, -22.4821) (-17.965, -22.4826) (-17.9499, -22.483) (-17.9349, -22.4833) (-17.9198, -22.4836) (-17.9048, -22.4837) (-17.8898, -22.4838) (-17.8749, -22.4839) (-17.8599, -22.4838) (-17.845, -22.4837) (-17.8301, -22.4835) (-17.8152, -22.4832) (-17.8004, -22.4829) (-17.7856, -22.4825) (-17.7708, -22.482) (-17.756, -22.4814) (-17.7413, -22.4807) (-17.7266, -22.48) (-17.7119, -22.4792) (-17.6973, -22.4783) (-17.6827, -22.4773) (-17.6681, -22.4762) (-17.6536, -22.4751) (-17.639, -22.4738) (-17.6246, -22.4725) (-17.6101, -22.4711) (-17.5957, -22.4696) (-17.5813, -22.4681) (-17.5669, -22.4664) (-17.5526, -22.4647) (-17.5384, -22.4628) (-17.5241, -22.4609) (-17.5099, -22.4589) (-17.4957, -22.4568) (-17.4816, -22.4545) (-17.4675, -22.4522) (-17.4535, -22.4498) (-17.4395, -22.4473) (-17.4256, -22.4447) (-17.4117, -22.442) (-17.3978, -22.4391) (-17.384, -22.4362) (-17.3702, -22.4332) (-17.3565, -22.4301) (-17.3428, -22.4268) (-17.3292, -22.4235) (-17.3157, -22.4199) (-17.3022, -22.4162) (-17.2888, -22.4123) (-17.2755, -22.4083) (-17.2623, -22.4042) (-17.249, -22.4) (-17.2359, -22.3957) (-17.2228, -22.3913) (-17.2098, -22.3867) (-17.1969, -22.3817) (-17.1869, -22.3773) (-17.1794, -22.3738) (-17.1745, -22.3713) (-17.1721, -22.3701) knots -1 -1 -1 -1 -1 -1 -0.98571429 -0.97142857 -0.95714286 -0.94285714 -0.92857143 -0.91428571 -0.9 -0.88571429 -0.87142857 -0.85714286 -0.84285714 -0.82857143 -0.81428571 -0.8 -0.78571429 -0.77142857 -0.75714286 -0.74285714 -0.72857143 -0.71428571 -0.7 -0.68571429 -0.67142857 -0.65714286 -0.64285714 -0.62857143 -0.61428571 -0.6 -0.58571429 -0.57142857 -0.55714286 -0.54285714 -0.52857143 -0.51428571 -0.5 -0.48571429 -0.47142857 -0.45714286 -0.44285714 -0.42857143 -0.41428571 -0.4 -0.38571429 -0.37142857 -0.35714286 -0.34285714 -0.32857143 -0.31428571 -0.3 -0.28571429 -0.27142857 -0.25714286 -0.24285714 -0.22857143 -0.21428571 -0.2 -0.18571429 -0.17142857 -0.15714286 -0.14285714 -0.12857143 -0.11428571 -0.1 -0.08571429 -0.07142857 -0.05714286 -0.04285714 -0.02857143 -0.01428571 0 0 0 0 0 0
  line L25 (-17.1721, -22.3701) -> (-17.1113, -22.3385)
  arc A51 (-16.7794, -22.4358) -> (-17.1113, -22.3385) centre (-16.9961, -22.5604) ccw
  arc A52 (-16.7794, -22.4358) -> (-16.721, -22.5351) centre (-11.6741, -19.5) ccw
  arc A53 (-16.7972, -22.8725) -> (-16.721, -22.5351) centre (-16.9352, -22.664) ccw
  line L26 (-16.7972, -22.8725) -> (-16.8544, -22.9103)
  spline S26 degree 5 poles (-16.8544, -22.9103) (-16.8566, -22.9118) (-16.8612, -22.9149) (-16.8679, -22.9197) (-16.8766, -22.9263) (-16.8872, -22.9351) (-16.8976, -22.9443) (-16.9078, -22.9536) (-16.9179, -22.963) (-16.928, -22.9725) (-16.9381, -22.9821) (-16.948, -22.9918) (-16.9579, -23.0016) (-16.9677, -23.0115) (-16.9774, -23.0217) (-16.9869, -23.0319) (-16.9964, -23.0423) (-17.0058, -23.0528) (-17.0151, -23.0633) (-17.0244, -23.074) (-17.0336, -23.0847) (-17.0428, -23.0955) (-17.0518, -23.1064) (-17.0608, -23.1175) (-17.0698, -23.1286) (-17.0786, -23.1397) (-17.0874, -23.151) (-17.0961, -23.1624) (-17.1048, -23.1738) (-17.1134, -23.1853) (-17.122, -23.1969) (-17.1305, -23.2086) (-17.1389, -23.2203) (-17.1472, -23.2321) (-17.1556, -23.244) (-17.1638, -23.2559) (-17.172, -23.2679) (-17.1801, -23.28) (-17.1882, -23.2922) (-17.1962, -23.3044) (-17.2042, -23.3167) (-17.2121, -23.3291) (-17.2199, -23.3415) (-17.2277, -23.354) (-17.2354, -23.3665) (-17.2431, -23.3792) (-17.2507, -23.3918) (-17.2583, -23.4046) (-17.2658, -23.4174) (-17.2733, -23.4302) (-17.2807, -23.4432) (-17.2881, -23.4561) (-17.2954, -23.4692) (-17.3026, -23.4823) (-17.3098, -23.4954) (-17.3169, -23.5086) (-17.324, -23.5219) (-17.331, -23.5352) (-17.338, -23.5486) (-17.345, -23.562) (-17.3518, -23.5755) (-17.3587, -23.589) (-17.3654, -23.6026) (-17.3721, -23.6163) (-17.3788, -23.63) (-17.3854, -23.6437) (-17.392, -23.6575) (-17.3985, -23.6714) (-17.4049, -23.6853) (-17.4113, -23.6993) (-17.4177, -23.7133) (-17.4227, -23.7245) (-17.4265, -23.733) (-17.429, -23.7386) (-17.4302, -23.7414) knots 0 0 0 0 0 0 0.01428571 0.02857143 0.04285714 0.05714286 0.07142857 0.08571429 0.1 0.11428571 0.12857143 0.14285714 0.15714286 0.17142857 0.18571429 0.2 0.21428571 0.22857143 0.24285714 0.25714286 0.27142857 0.28571429 0.3 0.31428571 0.32857143 0.34285714 0.35714286 0.37142857 0.38571429 0.4 0.41428571 0.42857143 0.44285714 0.45714286 0.47142857 0.48571429 0.5 0.51428571 0.52857143 0.54285714 0.55714286 0.57142857 0.58571429 0.6 0.61428571 0.62857143 0.64285714 0.65714286 0.67142857 0.68571429 0.7 0.71428571 0.72857143 0.74285714 0.75714286 0.77142857 0.78571429 0.8 0.81428571 0.82857143 0.84285714 0.85714286 0.87142857 0.88571429 0.9 0.91428571 0.92857143 0.94285714 0.95714286 0.97142857 0.98571429 1 1 1 1 1 1
  arc A54 (-17.4302, -23.7414) -> (-17.1882, -24.0517) centre (-11.6741, -19.5) ccw
  spline S27 degree 5 poles (-17.1882, -24.0517) (-17.1851, -24.0512) (-17.1791, -24.0501) (-17.1699, -24.0485) (-17.1578, -24.0464) (-17.1427, -24.0436) (-17.1276, -24.0408) (-17.1125, -24.0379) (-17.0975, -24.035) (-17.0825, -24.032) (-17.0676, -24.0289) (-17.0527, -24.0258) (-17.0378, -24.0226) (-17.023, -24.0193) (-17.0082, -24.016) (-16.9934, -24.0126) (-16.9787, -24.0091) (-16.964, -24.0056) (-16.9494, -24.002) (-16.9348, -23.9984) (-16.9203, -23.9947) (-16.9057, -23.9909) (-16.8913, -23.9871) (-16.8769, -23.9832) (-16.8625, -23.9792) (-16.8482, -23.9751) (-16.8339, -23.971) (-16.8196, -23.9668) (-16.8054, -23.9626) (-16.7913, -23.9583) (-16.7772, -23.9539) (-16.7631, -23.9495) (-16.7491, -23.9449) (-16.7351, -23.9403) (-16.7212, -23.9357) (-16.7074, -23.931) (-16.6936, -23.9262) (-16.6798, -23.9213) (-16.6661, -23.9163) (-16.6524, -23.9113) (-16.6388, -23.9062) (-16.6253, -23.9011) (-16.6118, -23.8958) (-16.5984, -23.8905) (-16.585, -23.8851) (-16.5717, -23.8796) (-16.5584, -23.8741) (-16.5453, -23.8685) (-16.5321, -23.8627) (-16.519, -23.857) (-16.506, -23.8511) (-16.4931, -23.8451) (-16.4802, -23.8391) (-16.4674, -23.8329) (-16.4547, -23.8267) (-16.4421, -23.8204) (-16.4295, -23.814) (-16.417, -23.8075) (-16.4045, -23.8009) (-16.3921, -23.7943) (-16.3799, -23.7875) (-16.3677, -23.7806) (-16.3557, -23.7735) (-16.3438, -23.7663) (-16.3319, -23.759) (-16.3202, -23.7516) (-16.3085, -23.7441) (-16.2969, -23.7365) (-16.2854, -23.7289) (-16.274, -23.721) (-16.2629, -23.7129) (-16.2543, -23.7061) (-16.248, -23.7007) (-16.2439, -23.6971) (-16.2419, -23.6952) knots -1 -1 -1 -1 -1 -1 -0.98571429 -0.97142857 -0.95714286 -0.94285714 -0.92857143 -0.91428571 -0.9 -0.88571429 -0.87142857 -0.85714286 -0.84285714 -0.82857143 -0.81428571 -0.8 -0.78571429 -0.77142857 -0.75714286 -0.74285714 -0.72857143 -0.71428571 -0.7 -0.68571429 -0.67142857 -0.65714286 -0.64285714 -0.62857143 -0.61428571 -0.6 -0.58571429 -0.57142857 -0.55714286 -0.54285714 -0.52857143 -0.51428571 -0.5 -0.48571429 -0.47142857 -0.45714286 -0.44285714 -0.42857143 -0.41428571 -0.4 -0.38571429 -0.37142857 -0.35714286 -0.34285714 -0.32857143 -0.31428571 -0.3 -0.28571429 -0.27142857 -0.25714286 -0.24285714 -0.22857143 -0.21428571 -0.2 -0.18571429 -0.17142857 -0.15714286 -0.14285714 -0.12857143 -0.11428571 -0.1 -0.08571429 -0.07142857 -0.05714286 -0.04285714 -0.02857143 -0.01428571 0 0 0 0 0 0
  line L27 (-16.2419, -23.6952) -> (-16.1913, -23.649)
  arc A55 (-15.8456, -23.6571) -> (-16.1913, -23.649) centre (-16.0227, -23.8336) ccw
  arc A56 (-15.8456, -23.6571) -> (-15.7635, -23.7379) centre (-11.6741, -19.5) ccw
  arc A57 (-15.7498, -24.0835) -> (-15.7635, -23.7379) centre (-15.9371, -23.9178) ccw
  line L28 (-15.7498, -24.0835) -> (-15.7952, -24.1348)
  spline S28 degree 5 poles (-15.7952, -24.1348) (-15.797, -24.1369) (-15.8006, -24.141) (-15.8058, -24.1474) (-15.8125, -24.1561) (-15.8205, -24.1673) (-15.8281, -24.1788) (-15.8356, -24.1904) (-15.843, -24.2022) (-15.8503, -24.214) (-15.8575, -24.2258) (-15.8646, -24.2378) (-15.8716, -24.2498) (-15.8785, -24.262) (-15.8852, -24.2742) (-15.8918, -24.2866) (-15.8983, -24.2991) (-15.9046, -24.3116) (-15.9109, -24.3243) (-15.9171, -24.337) (-15.9232, -24.3497) (-15.9292, -24.3625) (-15.9352, -24.3754) (-15.941, -24.3884) (-15.9468, -24.4014) (-15.9524, -24.4145) (-15.958, -24.4277) (-15.9635, -24.4409) (-15.9689, -24.4542) (-15.9743, -24.4675) (-15.9795, -24.4809) (-15.9847, -24.4944) (-15.9898, -24.5079) (-15.9948, -24.5215) (-15.9998, -24.5351) (-16.0046, -24.5488) (-16.0094, -24.5625) (-16.0142, -24.5763) (-16.0188, -24.5901) (-16.0234, -24.604) (-16.0279, -24.6179) (-16.0323, -24.6319) (-16.0367, -24.646) (-16.041, -24.66) (-16.0452, -24.6742) (-16.0494, -24.6883) (-16.0534, -24.7026) (-16.0575, -24.7168) (-16.0614, -24.7311) (-16.0653, -24.7455) (-16.0691, -24.7599) (-16.0728, -24.7743) (-16.0765, -24.7888) (-16.0801, -24.8033) (-16.0837, -24.8179) (-16.0871, -24.8325) (-16.0906, -24.8471) (-16.0939, -24.8618) (-16.0972, -24.8766) (-16.1004, -24.8913) (-16.1035, -24.9061) (-16.1066, -24.921) (-16.1097, -24.9359) (-16.1126, -24.9508) (-16.1155, -24.9657) (-16.1183, -24.9807) (-16.1211, -24.9958) (-16.1238, -25.0108) (-16.1264, -25.0259) (-16.129, -25.0411) (-16.1315, -25.0562) (-16.1335, -25.0684) (-16.1349, -25.0775) (-16.1359, -25.0836) (-16.1363, -25.0867) knots 0 0 0 0 0 0 0.01428571 0.02857143 0.04285714 0.05714286 0.07142857 0.08571429 0.1 0.11428571 0.12857143 0.14285714 0.15714286 0.17142857 0.18571429 0.2 0.21428571 0.22857143 0.24285714 0.25714286 0.27142857 0.28571429 0.3 0.31428571 0.32857143 0.34285714 0.35714286 0.37142857 0.38571429 0.4 0.41428571 0.42857143 0.44285714 0.45714286 0.47142857 0.48571429 0.5 0.51428571 0.52857143 0.54285714 0.55714286 0.57142857 0.58571429 0.6 0.61428571 0.62857143 0.64285714 0.65714286 0.67142857 0.68571429 0.7 0.71428571 0.72857143 0.74285714 0.75714286 0.77142857 0.78571429 0.8 0.81428571 0.82857143 0.84285714 0.85714286 0.87142857 0.88571429 0.9 0.91428571 0.92857143 0.94285714 0.95714286 0.97142857 0.98571429 1 1 1 1 1 1
  arc A58 (-16.1363, -25.0867) -> (-15.8222, -25.3237) centre (-11.6741, -19.5) ccw
  spline S29 degree 5 poles (-15.8222, -25.3237) (-15.8194, -25.3224) (-15.8138, -25.3199) (-15.8054, -25.316) (-15.7943, -25.3107) (-15.7804, -25.3042) (-15.7665, -25.2975) (-15.7527, -25.2908) (-15.739, -25.2841) (-15.7253, -25.2773) (-15.7116, -25.2705) (-15.698, -25.2636) (-15.6845, -25.2567) (-15.671, -25.2497) (-15.6576, -25.2426) (-15.6442, -25.2356) (-15.6309, -25.2284) (-15.6176, -25.2212) (-15.6044, -25.214) (-15.5913, -25.2067) (-15.5782, -25.1993) (-15.5652, -25.1919) (-15.5522, -25.1845) (-15.5393, -25.177) (-15.5264, -25.1694) (-15.5136, -25.1618) (-15.5009, -25.1541) (-15.4882, -25.1464) (-15.4756, -25.1386) (-15.463, -25.1308) (-15.4505, -25.1229) (-15.4381, -25.115) (-15.4257, -25.107) (-15.4134, -25.0989) (-15.4012, -25.0908) (-15.3891, -25.0827) (-15.377, -25.0745) (-15.3649, -25.0662) (-15.353, -25.0579) (-15.3411, -25.0495) (-15.3293, -25.0411) (-15.3175, -25.0326) (-15.3058, -25.024) (-15.2943, -25.0154) (-15.2827, -25.0067) (-15.2713, -24.998) (-15.2599, -24.9892) (-15.2486, -24.9803) (-15.2374, -24.9714) (-15.2263, -24.9625) (-15.2152, -24.9534) (-15.2043, -24.9443) (-15.1934, -24.9351) (-15.1827, -24.9259) (-15.172, -24.9166) (-15.1614, -24.9072) (-15.1509, -24.8978) (-15.1405, -24.8883) (-15.1302, -24.8787) (-15.1199, -24.869) (-15.1098, -24.8593) (-15.0999, -24.8495) (-15.0901, -24.8395) (-15.0804, -24.8295) (-15.0709, -24.8194) (-15.0615, -24.8092) (-15.0521, -24.7989) (-15.0429, -24.7886) (-15.0337, -24.7783) (-15.0248, -24.7677) (-15.0162, -24.757) (-15.0096, -24.7482) (-15.0049, -24.7414) (-15.0019, -24.7368) (-15.0004, -24.7345) knots -1 -1 -1 -1 -1 -1 -0.98571429 -0.97142857 -0.95714286 -0.94285714 -0.92857143 -0.91428571 -0.9 -0.88571429 -0.87142857 -0.85714286 -0.84285714 -0.82857143 -0.81428571 -0.8 -0.78571429 -0.77142857 -0.75714286 -0.74285714 -0.72857143 -0.71428571 -0.7 -0.68571429 -0.67142857 -0.65714286 -0.64285714 -0.62857143 -0.61428571 -0.6 -0.58571429 -0.57142857 -0.55714286 -0.54285714 -0.52857143 -0.51428571 -0.5 -0.48571429 -0.47142857 -0.45714286 -0.44285714 -0.42857143 -0.41428571 -0.4 -0.38571429 -0.37142857 -0.35714286 -0.34285714 -0.32857143 -0.31428571 -0.3 -0.28571429 -0.27142857 -0.25714286 -0.24285714 -0.22857143 -0.21428571 -0.2 -0.18571429 -0.17142857 -0.15714286 -0.14285714 -0.12857143 -0.11428571 -0.1 -0.08571429 -0.07142857 -0.05714286 -0.04285714 -0.02857143 -0.01428571 0 0 0 0 0 0
  line L29 (-15.0004, -24.7345) -> (-14.9636, -24.6768)
  arc A59 (-14.6275, -24.5951) -> (-14.9636, -24.6768) centre (-14.7529, -24.8114) ccw
  arc A60 (-14.6275, -24.5951) -> (-14.5273, -24.6519) centre (-11.6741, -19.5) ccw
  arc A61 (-14.4246, -24.9822) -> (-14.5273, -24.6519) centre (-14.6484, -24.8706) ccw
  line L30 (-14.4246, -24.9822) -> (-14.4552, -25.0435)
  spline S30 degree 5 poles (-14.4552, -25.0435) (-14.4564, -25.0459) (-14.4588, -25.0509) (-14.4622, -25.0584) (-14.4664, -25.0685) (-14.4712, -25.0814) (-14.4756, -25.0945) (-14.4798, -25.1077) (-14.4839, -25.1209) (-14.4879, -25.1342) (-14.4918, -25.1475) (-14.4956, -25.1609) (-14.4992, -25.1744) (-14.5027, -25.1879) (-14.5061, -25.2015) (-14.5092, -25.2151) (-14.5122, -25.2288) (-14.5151, -25.2426) (-14.5179, -25.2564) (-14.5206, -25.2703) (-14.5232, -25.2842) (-14.5257, -25.2981) (-14.5281, -25.3121) (-14.5304, -25.3262) (-14.5326, -25.3402) (-14.5347, -25.3544) (-14.5367, -25.3685) (-14.5385, -25.3827) (-14.5403, -25.3969) (-14.542, -25.4112) (-14.5436, -25.4255) (-14.5452, -25.4399) (-14.5466, -25.4542) (-14.5479, -25.4686) (-14.5492, -25.4831) (-14.5504, -25.4976) (-14.5514, -25.5121) (-14.5524, -25.5266) (-14.5533, -25.5412) (-14.5542, -25.5558) (-14.5549, -25.5704) (-14.5556, -25.585) (-14.5562, -25.5997) (-14.5567, -25.6144) (-14.5571, -25.6292) (-14.5574, -25.6439) (-14.5577, -25.6587) (-14.5579, -25.6735) (-14.558, -25.6884) (-14.558, -25.7033) (-14.558, -25.7182) (-14.5579, -25.7331) (-14.5577, -25.748) (-14.5574, -25.763) (-14.557, -25.778) (-14.5566, -25.793) (-14.5561, -25.808) (-14.5556, -25.823) (-14.5549, -25.8381) (-14.5542, -25.8532) (-14.5534, -25.8683) (-14.5525, -25.8835) (-14.5516, -25.8986) (-14.5506, -25.9138) (-14.5495, -25.929) (-14.5484, -25.9442) (-14.5472, -25.9595) (-14.5459, -25.9747) (-14.5445, -25.99) (-14.5431, -26.0053) (-14.5416, -26.0206) (-14.5403, -26.0328) (-14.5394, -26.042) (-14.5387, -26.0482) (-14.5384, -26.0512) knots 0 0 0 0 0 0 0.01428571 0.02857143 0.04285714 0.05714286 0.07142857 0.08571429 0.1 0.11428571 0.12857143 0.14285714 0.15714286 0.17142857 0.18571429 0.2 0.21428571 0.22857143 0.24285714 0.25714286 0.27142857 0.28571429 0.3 0.31428571 0.32857143 0.34285714 0.35714286 0.37142857 0.38571429 0.4 0.41428571 0.42857143 0.44285714 0.45714286 0.47142857 0.48571429 0.5 0.51428571 0.52857143 0.54285714 0.55714286 0.57142857 0.58571429 0.6 0.61428571 0.62857143 0.64285714 0.65714286 0.67142857 0.68571429 0.7 0.71428571 0.72857143 0.74285714 0.75714286 0.77142857 0.78571429 0.8 0.81428571 0.82857143 0.84285714 0.85714286 0.87142857 0.88571429 0.9 0.91428571 0.92857143 0.94285714 0.95714286 0.97142857 0.98571429 1 1 1 1 1 1
  arc A62 (-14.5384, -26.0512) -> (-14.1736, -26.1989) centre (-11.6741, -19.5) ccw
  spline S31 degree 5 poles (-14.1736, -26.1989) (-14.1712, -26.1969) (-14.1665, -26.193) (-14.1594, -26.187) (-14.1499, -26.1791) (-14.1382, -26.1692) (-14.1266, -26.1592) (-14.115, -26.1491) (-14.1034, -26.1391) (-14.092, -26.129) (-14.0805, -26.1189) (-14.0692, -26.1087) (-14.0579, -26.0985) (-14.0467, -26.0882) (-14.0356, -26.078) (-14.0245, -26.0677) (-14.0135, -26.0573) (-14.0025, -26.0469) (-13.9916, -26.0365) (-13.9808, -26.0261) (-13.9701, -26.0156) (-13.9594, -26.005) (-13.9488, -25.9945) (-13.9383, -25.9839) (-13.9278, -25.9733) (-13.9174, -25.9626) (-13.9071, -25.9519) (-13.8968, -25.9411) (-13.8867, -25.9304) (-13.8766, -25.9196) (-13.8665, -25.9087) (-13.8566, -25.8978) (-13.8467, -25.8869) (-13.8369, -25.876) (-13.8272, -25.865) (-13.8176, -25.8539) (-13.808, -25.8429) (-13.7985, -25.8318) (-13.7891, -25.8206) (-13.7798, -25.8095) (-13.7706, -25.7983) (-13.7614, -25.787) (-13.7524, -25.7757) (-13.7434, -25.7644) (-13.7345, -25.753) (-13.7257, -25.7417) (-13.717, -25.7302) (-13.7084, -25.7187) (-13.6999, -25.7072) (-13.6915, -25.6957) (-13.6831, -25.6841) (-13.6749, -25.6725) (-13.6668, -25.6608) (-13.6588, -25.6491) (-13.6509, -25.6373) (-13.6431, -25.6255) (-13.6354, -25.6137) (-13.6278, -25.6018) (-13.6203, -25.5899) (-13.6129, -25.5779) (-13.6057, -25.5659) (-13.5986, -25.5539) (-13.5917, -25.5417) (-13.585, -25.5295) (-13.5784, -25.5173) (-13.572, -25.505) (-13.5656, -25.4927) (-13.5593, -25.4803) (-13.5532, -25.4679) (-13.5472, -25.4555) (-13.5417, -25.4429) (-13.5376, -25.4327) (-13.5349, -25.4249) (-13.5331, -25.4197) (-13.5323, -25.4171) knots -1 -1 -1 -1 -1 -1 -0.98571429 -0.97142857 -0.95714286 -0.94285714 -0.92857143 -0.91428571 -0.9 -0.88571429 -0.87142857 -0.85714286 -0.84285714 -0.82857143 -0.81428571 -0.8 -0.78571429 -0.77142857 -0.75714286 -0.74285714 -0.72857143 -0.71428571 -0.7 -0.68571429 -0.67142857 -0.65714286 -0.64285714 -0.62857143 -0.61428571 -0.6 -0.58571429 -0.57142857 -0.55714286 -0.54285714 -0.52857143 -0.51428571 -0.5 -0.48571429 -0.47142857 -0.45714286 -0.44285714 -0.42857143 -0.41428571 -0.4 -0.38571429 -0.37142857 -0.35714286 -0.34285714 -0.32857143 -0.31428571 -0.3 -0.28571429 -0.27142857 -0.25714286 -0.24285714 -0.22857143 -0.21428571 -0.2 -0.18571429 -0.17142857 -0.15714286 -0.14285714 -0.12857143 -0.11428571 -0.1 -0.08571429 -0.07142857 -0.05714286 -0.04285714 -0.02857143 -0.01428571 0 0 0 0 0 0
  line L31 (-13.5323, -25.4171) -> (-13.5116, -25.3518)
  arc A63 (-13.2082, -25.1859) -> (-13.5116, -25.3518) centre (-13.2733, -25.4273) ccw
  arc A64 (-13.2082, -25.1859) -> (-13.0966, -25.2148) centre (-11.6741, -19.5) ccw
  arc A65 (-12.912, -25.5073) -> (-13.0966, -25.2148) centre (-13.157, -25.4574) ccw
  line L32 (-12.912, -25.5073) -> (-12.9257, -25.5744)